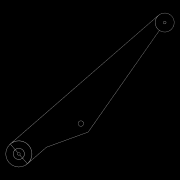
# Autodesk Inventor part: large-upper-arm
Saved by Autodesk Inventor 2020 (Build 240168000, 168)
## iProperties
Created: 2020-03-24
Part Number: large-upper-arm
Material: Generic
Document SubType Name: Modeling
Designer: valer
Density: 1 g/cm^3
Appearance: Default
Mass: 1308.33 g
Surface Area: 1161.01 cm^2
Volume: 1308.33 cm^3
Author: valer
Autodesk Inventor part; units mm, degrees
ref_plane "YZ Plane" through (0, 0, 0) normal (1, 0, 0) x (0, 1, 0)
ref_plane "XZ Plane" through (0, 0, 0) normal (0, 1, 0) x (-1, 0, 0)
ref_plane "XY Plane" through (0, 0, 0) normal (0, 0, 1) x (1, 0, 0)
sketch "Body" plane through (0, 0, 0) normal (0, 0, 1) x (1, 0, 0)
  circle A0 centre (0, 0) radius 12.7
  line L0 (0, 0) -> (330.3279, 297.4286) construction
  line L1 (-105.9436, 0) -> (428.2281, 0) projected
  circle A1 centre (330.3279, 297.4286) radius 12.7
  circle A2 centre (0, 0) radius 29.6333
  circle A3 centre (330.3279, 297.4286) radius 21.59
  line L2 (316.174, 313.7318) -> (-19.4268, 22.3771)
  line L3 (157.0944, 49.4885) -> (94.651, 121.4147) construction
  line L4 (19.4268, -22.3771) -> (62.5826, 15.089)
  line L5 (62.5826, 15.089) -> (157.0944, 49.4885)
  line L6 (62.5826, 15.089) -> (23.7289, 59.8431) construction
  line L7 (157.0944, 49.4885) -> (318.198, 279.5682)
  circle A4 centre (140.4428, 68.6688) radius 6.35
  line L8 (140.4428, 68.6688) -> (330.3279, 297.4286) construction
  circle A5 centre (249.2132, 199.7075) radius 3.175
  circle A6 centre (51.0855, 57.3906) radius 3.175
  line L9 (51.0855, 57.3906) -> (43.8157, 19.9906) construction
  circle A7 centre (43.8157, 19.9906) radius 3.175
  line L10 (47.9688, 57.9964) -> (40.699, 20.5964)
  line L11 (54.2021, 56.7848) -> (46.9323, 19.3848)
  line L12 (69.7252, 73.4134) -> (61.4861, 31.0268) construction
  line L13 (66.6086, 74.0192) -> (58.3694, 31.6326)
  line L14 (64.6028, 30.4209) -> (72.8419, 72.8076)
  arc A8 (72.8419, 72.8076) -> (66.6086, 74.0192) centre (69.7252, 73.4134) ccw
  arc A9 (58.3694, 31.6326) -> (64.6028, 30.4209) centre (61.4861, 31.0268) ccw
  line L15 (51.0855, 57.3906) -> (330.3279, 297.4286) construction
  line L16 (91.4716, 92.1067) -> (82.2632, 44.7334) construction
  line L17 (91.4716, 92.1067) -> (82.2632, 44.7334) construction
  line L18 (88.355, 92.7125) -> (79.1465, 45.3392)
  line L19 (85.3799, 44.1276) -> (94.5883, 91.5009)
  arc A10 (94.5883, 91.5009) -> (88.355, 92.7125) centre (91.4716, 92.1067) ccw
  arc A11 (79.1465, 45.3392) -> (85.3799, 44.1276) centre (82.2632, 44.7334) ccw
  line L20 (113.218, 110.8) -> (103.0403, 58.44) construction
  line L21 (113.218, 110.8) -> (103.0403, 58.44) construction
  line L22 (110.1014, 111.4058) -> (99.9236, 59.0458)
  line L23 (106.1569, 57.8342) -> (116.3347, 110.1942)
  arc A12 (116.3347, 110.1942) -> (110.1014, 111.4058) centre (113.218, 110.8) ccw
  arc A13 (99.9236, 59.0458) -> (106.1569, 57.8342) centre (103.0403, 58.44) ccw
  line L24 (134.9644, 129.4933) -> (123.8173, 72.1466) construction
  line L25 (131.8477, 130.0991) -> (120.7007, 72.7524)
  line L26 (126.934, 71.5408) -> (138.0811, 128.8875)
  arc A14 (138.0811, 128.8875) -> (131.8477, 130.0991) centre (134.9644, 129.4933) ccw
  arc A15 (120.7007, 72.7524) -> (126.934, 71.5408) centre (123.8173, 72.1466) ccw
  line L27 (321.0449, 306.0955) -> (129.3909, 100.82) construction
  line L28 (179.3056, 154.2823) -> (292.8806, 275.9294) construction
  line L29 (181.6264, 152.1156) -> (295.2013, 273.7627)
  line L30 (290.5598, 278.0962) -> (176.9849, 156.4491)
  arc A16 (176.9849, 156.4491) -> (181.6264, 152.1156) centre (179.3056, 154.2823) ccw
  arc A17 (295.2013, 273.7627) -> (290.5598, 278.0962) centre (292.8806, 275.9294) ccw
  line L31 (179.3056, 154.2823) -> (198.3712, 138.4567) construction
  line L32 (191.8565, 143.8643) -> (224.3023, 182.9528) construction
  line L33 (189.4134, 145.8922) -> (221.8593, 184.9806)
  line L34 (226.7454, 180.9249) -> (194.2995, 141.8365)
  arc A18 (189.4134, 145.8922) -> (194.2995, 141.8365) centre (191.8565, 143.8643) ccw
  arc A19 (226.7454, 180.9249) -> (221.8593, 184.9806) centre (224.3023, 182.9528) ccw
  circle A20 centre (0, 0) radius 3.175
  circle A21 centre (330.3279, 297.4286) radius 3.175
  point P0 (65.6057, 52.2201)
  point P1 (86.8674, 68.42)
  point P2 (108.1291, 84.62)
  point P3 (236.0931, 215.1059)
  point P4 (208.0794, 163.4086)
  point P5 (29.6333, 0)
  point P6 (45.2021, 0)
  dimension "d26" = 25.4
  dimension "d23" = 25.4
  dimension "d24" = 42
  dimension "d27" = 59.2667
  dimension "d28" = 43.18
  dimension "d29" = 95.25
  dimension "d30" = 444.5
  dimension "d31" = 57.15
  dimension "d32" = 22
  dimension "d34" = 13
  dimension "d35" = 12.7
  dimension "d36" = 25.4
  dimension "d37" = 6.35
  dimension "d38" = 127
  dimension "d39" = 6.35
  dimension "d40" = 37
  dimension "d41" = 19.05
  dimension "d42" = 38.1
  dimension "d43" = 8.4667
  dimension "d44" = 15.24
  dimension "d45" = 43.18
  dimension "d46" = 48.26
  dimension "d47" = 17.78
  dimension "d48" = 53.34
  dimension "d49" = 17.78
  dimension "d50" = 17.78
  dimension "d51" = 58.42
  dimension "d52" = 43.18
  dimension "d53" = 50.8
  dimension "d54" = 8.4667
  dimension "d55" = 50.8
  dimension "d58" = 6.35
  dimension "d59" = 6.35
  constraints: 80 end point, 32 point on circle, 31 tangent, 21 centre point, 12 parallel, 12 point on line, 7 coincident, 7 equal radius, 6 midpoint, 3 perpendicular, 1 collinear, 4 other
  measures "d23" diameter of A0
  measures "d24" angle of L0 L1
  measures "d27" diameter of A2
  measures "d28" diameter of A3
  measures "d29" distance of L3.start L3.end
  measures "d30" distance of L0.start L0.end
  measures "d31" distance from line of point (0, 0) L6
  measures "d32" angle of L0 L5
  measures "d34" angle of L0 L7
  measures "d35" diameter of A4
  measures "d36" distance of L3.start L8.start
  measures "d37" diameter of A5
  measures "d38" distance of L0.end A5.centre
  measures "d39" diameter of A6
  measures "d40" angle of L0 L9
  measures "d41" distance from line of L6 L9.start
  measures "d42" distance of L9.start L9.end
  measures "d43" distance from line of L0 L9.start
  measures "d44" distance between parallel lines of L9 L12
  measures "d45" distance of L12.start L12.end
  measures "d46" distance of L16.start L16.end
  measures "d47" distance between parallel lines of L16 L12
  measures "d48" distance of L20.start L20.end
  measures "d49" distance between parallel lines of L20 L16
  measures "d50" distance between parallel lines of L20 L24
  measures "d51" distance of L24.start L24.end
  measures "d52" distance of L0.end L28.end
  measures "d53" distance of L24.start L28.start
  measures "d54" distance between parallel lines of L8 L32
  measures "d55" distance of L32.start L32.end
  measures "d58" diameter of A20
  measures "d59" diameter of A21
extrude "BodyFeature" add sketch "Body" along normal mid plane 50.8 contours L1 A20 A0 | L1 A2 A0 | A0 L1 A20 | A0 L1 A2 | A2 L2 A3 L7 L5 L4 L1 | L1 L4 A2 | A3 | A1 | A5 | A6 | A6 L11 A7 L10 | A7 | A8 L14 A9 L13 | A10 L19 A11 L18 | A12 L23 A13 L22 | A14 L26 A15 L25 | A16 L30 A17 L29 | L33 A19 L34 A18 | A21
extrude "BodyMountFeature" add sketch "Body" along normal mid plane 63.5 contours L1 A2 A0 | A0 L1 A2
sketch "BodySculpt" plane through (-19.4268, 22.3771, 25.4) normal (-0.6555737, 0.7551312, 0) x (0.7551312, 0.6555737, 0)
  line L0 (0, 50.8) -> (0, 0) projected
  line L1 (466.0172, 50.8) -> (466.0172, 0) projected
  line L2 (444.4272, 0) -> (0, 0) projected
  line L3 (0, 0) -> (466.0172, 10.1685)
  line L4 (466.0172, 10.1685) -> (466.0172, 40.6315)
  line L5 (466.0172, 40.6315) -> (0, 50.8)
  line L6 (0, 50.8) -> (444.4272, 50.8) projected
  line L7 (-29.6333, -6.35) -> (29.6333, -6.35) projected
  line L8 (29.6333, 57.15) -> (-29.6333, 57.15) projected
  line L9 (0, 0) -> (0, 50.8) projected
  line L10 (0, 0) -> (0, 0) projected
  line L11 (0, 50.8) -> (0, 0) projected
  line L12 (0, 50.8) -> (0, 50.8) projected
  line L13 (-29.6333, 57.15) -> (-29.6333, -6.35) projected
  line L14 (29.6333, -6.35) -> (29.6333, 57.15)
  point P0 (0, 25.4)
  point P1 (29.6333, 0)
  point P2 (29.6333, 50.8)
  dimension "d62" = 1.25
  dimension "d63" = 1.25
  constraints: 8 end point, 1 collinear, 1 perpendicular
  measures "d62" angle of L2 L3
  measures "d63" angle of L6 L5
extrude "BodySculptFeature" cut sketch "BodySculpt" against normal through all contours L5 L14 L3 L0 | L0 L2 L14 L7 L13 L8 L6 | L5 L1 L3 L14 keep common part
extrude "ForearmMountFeature" add sketch "Body" along normal mid plane 38.1 contours A3 | A1
body "Solid2"
